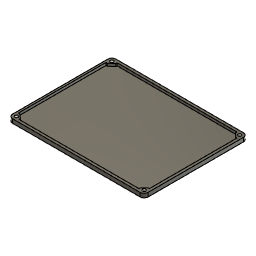
PCB_CASE_PART_2 v2 (Autodesk Fusion 360 design; units mm, degrees)
Autodesk Fusion 360 part; units mm, degrees
sketch "Sketch1" plane through (0, 0, 0) normal (0, 1, 0) x (1, 0, 0)
  line L0 (0, 0) -> (103, 0)
  line L1 (103, 0) -> (103, 78.5)
  line L2 (103, 78.5) -> (0, 78.5)
  line L3 (0, 78.5) -> (0, 0)
  dimension "d1" = 103
  dimension "d2" = 78.5
  constraint horizontal L0
  constraint vertical L1
  constraint horizontal L2
  constraint vertical L3
  constraint coincident L0.start L3.end
  measures "d1" distance of L1.end L2.end
  measures "d2" distance of L0.end L1.end
extrude "Extrude1" add sketch "Sketch1" along normal blind 3
fillet "Fillet1" radius 3 4 edges at (0, 1.5, 0) (103, 1.5, 0) (103, 1.5, -78.5) (0, 1.5, -78.5)
sketch "Sketch6" plane through (0, 3, 0) normal (0, 1, 0) x (-1, 0, 0)
  arc A0 (-3, -78.5) -> (0, -75.5) centre (-3, -75.5) ccw
  line L0 (0, -75.5) -> (0, -3)
  arc A1 (0, -3) -> (-3, 0) centre (-3, -3) ccw
  line L1 (-3, 0) -> (-100, 0)
  arc A2 (-100, 0) -> (-103, -3) centre (-100, -3) ccw
  line L2 (-103, -3) -> (-103, -75.5)
  arc A3 (-103, -75.5) -> (-100, -78.5) centre (-100, -75.5) ccw
  line L3 (-100, -78.5) -> (-3, -78.5)
  line L4 (-1.5, -72.5) -> (-1.5, -6)
  line L5 (-1.5, -6) -> (-2.5, -6)
  line L6 (-2.5, -6) -> (-6, -3)
  line L7 (-6, -3) -> (-6, -2)
  line L8 (-6, -2) -> (-97, -2)
  line L9 (-97, -2) -> (-97, -3)
  line L10 (-97, -3) -> (-100, -6)
  line L11 (-100, -6) -> (-101, -6)
  line L12 (-101, -6) -> (-101, -72.5)
  line L13 (-101, -72.5) -> (-100, -72.5)
  line L14 (-100, -72.5) -> (-97, -75.5)
  line L15 (-97, -75.5) -> (-97, -76.5)
  line L16 (-97, -76.5) -> (-6, -76.5)
  line L17 (-6, -76.5) -> (-6.0056, -75.5)
  line L18 (-6.0056, -75.5) -> (-2.5, -72.4923)
  line L19 (-2.5, -72.4923) -> (-1.5, -72.5)
  dimension "d181" = 6
  dimension "d182" = 6
  dimension "d184" = 1
  dimension "d185" = 6
  dimension "d186" = 66.5
  dimension "d187" = 1
  dimension "d188" = 1
  dimension "d189" = 1
  dimension "d191" = 6
  dimension "d192" = 6
  dimension "d193" = 1
  dimension "d194" = 1
  dimension "d195" = 6
  dimension "d196" = 1
  dimension "d197" = 6
  dimension "d198" = 1
  dimension "d199" = 6
  dimension "d200" = 2
  dimension "d201" = 2
  dimension "d202" = 2
  dimension "d203" = 2
  dimension "d204" = 2
  dimension "d205" = 2
  dimension "d206" = 1.5
  dimension "d207" = 2
  constraint parallel L0 L4
  constraint perpendicular L5 L7
  constraint perpendicular L7 L8
  constraint perpendicular L8 L9
  constraint perpendicular L9 L11
  constraint perpendicular L12 L13
  constraint perpendicular L15 L16
  measures "d181" distance of L3 L4.start
  measures "d182" distance of L0 L16.end
  measures "d184" distance of L17.end L16.end
  measures "d185" distance of L1 L4.end
  measures "d186" distance of L4.end L4.start
  measures "d187" distance of L18.end L4.start
  measures "d188" distance of L4.end L5.end
  measures "d189" distance of L6.end L7.end
  measures "d191" distance of L0 L7.end
  measures "d192" distance of L2 L8.end
  measures "d193" distance of L8.end L9.end
  measures "d194" distance of L10.end L11.end
  measures "d195" distance of L1 L11.end
  measures "d196" distance of L12.end L13.end
  measures "d197" distance of L3 L12.end
  measures "d198" distance of L14.end L15.end
  measures "d199" distance of L2 L15.end
  measures "d200" distance of L3 L16.end
  measures "d201" distance of L3 L15.end
  measures "d202" distance of L2 L12.end
  measures "d203" distance of L2 L11.end
  measures "d204" distance of L1 L8.end
  measures "d205" distance of L1 L7.end
  measures "d206" distance of L0 L4.end
extrude "Extrude6" cut sketch "Sketch6" against normal blind 2 contours L4 L5 L6 L7 L8 L9 L10 L11 L12 L13 L14 L15 L16 L17 L18 L19
sketch "Sketch7" plane through (0, 3, 0) normal (0, 1, 0) x (-1, 0, 0)
  line L0 (-1.5, -6) -> (-1.5, -72.5)
  line L1 (-1.5, -72.5) -> (-2.5, -72.4923)
  line L2 (-2.5, -72.4923) -> (-6.0056, -75.5)
  line L3 (-6.0056, -75.5) -> (-6, -76.5)
  line L4 (-6, -76.5) -> (-97, -76.5)
  line L5 (-97, -76.5) -> (-97, -75.5)
  line L6 (-97, -75.5) -> (-100, -72.5)
  line L7 (-100, -72.5) -> (-101, -72.5)
  line L8 (-101, -72.5) -> (-101, -6)
  line L9 (-101, -6) -> (-100, -6)
  line L10 (-100, -6) -> (-97, -3)
  line L11 (-97, -3) -> (-97, -2)
  line L12 (-97, -2) -> (-6, -2)
  line L13 (-6, -2) -> (-6, -3)
  line L14 (-6, -3) -> (-2.5, -6)
  line L15 (-2.5, -6) -> (-1.5, -6)
  arc A0 (-3, -78.5) -> (0, -75.5) centre (-3, -75.5) ccw
  line L16 (0, -75.5) -> (0, -3)
  arc A1 (0, -3) -> (-3, 0) centre (-3, -3) ccw
  line L17 (-3, 0) -> (-100, 0)
  arc A2 (-100, 0) -> (-103, -3) centre (-100, -3) ccw
  line L18 (-103, -3) -> (-103, -75.5)
  arc A3 (-103, -75.5) -> (-100, -78.5) centre (-100, -75.5) ccw
  line L19 (-100, -78.5) -> (-3, -78.5)
  point P0 (-3, -75.5)
  point P1 (-100, -75.5)
  point P2 (-3, -3)
  point P3 (-100, -3)
  constraint coincident P0 A0.centre
  constraint coincident P1 A3.centre
  constraint coincident P2 A1.centre
  constraint coincident P3 A2.centre
hole "Hole1" at (3, 3, -75.5) at (100, 3, -75.5) at (3, 3, -3) at (100, 3, -3) direction (0, -1, 0) diameter 2.529 depth 2 tip angle 180
thread "Thread1" "ISO Metric profile 3.0 M3x0.5 6H"
